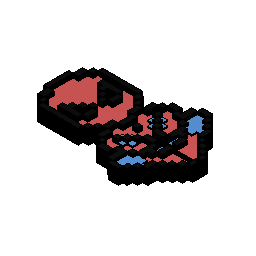
Spider-man v1 (Autodesk Fusion 360 design; units mm, degrees)
Autodesk Fusion 360 part; units mm, degrees
note: some values were not read from the file. Chosen so that the rebuilt part matches the saved one: which bodies a step acts on; which face or edge a step refers to. Set by a fixed rule: which sketch regions a step uses.
sketch "spider-man" plane through (0, 0, 0) normal (0, 0, 1) x (1, 0, 0)
  line L0 (48.5, 2.7143) -> (48.5, 6)
  line L1 (48.5, 6) -> (45.5, 6)
  line L2 (45.5, 6) -> (45.5, 9.5)
  line L3 (45.5, 9.5) -> (42, 9.5)
  line L4 (42, 9.5) -> (42, 13)
  line L5 (42, 13) -> (38.5, 13)
  line L6 (38.5, 13) -> (38.2383, 13)
  line L7 (38.2383, 13) -> (38.2383, 16)
  line L8 (38.2383, 16) -> (35, 16)
  line L9 (35, 16) -> (35, 23)
  line L10 (35, 23) -> (32, 23)
  line L11 (32, 23) -> (32, 26.5)
  line L12 (32, 26.5) -> (28.5, 26.5)
  line L13 (28.5, 26.5) -> (28.5, 30)
  line L14 (28.5, 30) -> (25, 30)
  line L15 (25, 30) -> (25, 33.5)
  line L16 (25, 33.5) -> (18, 33.5)
  line L17 (18, 33.5) -> (18, 30)
  line L18 (18, 30) -> (14, 30)
  line L19 (14, 30) -> (14, 23)
  line L20 (14, 23) -> (11, 23)
  line L21 (11, 23) -> (11, 26.5)
  line L22 (11, 26.5) -> (4.5, 26.5)
  line L23 (4.5, 26.5) -> (4.5, 23)
  line L24 (4.5, 23) -> (1, 23)
  line L25 (1, 23) -> (1, 20)
  line L26 (1, 20) -> (-2.5282, 20)
  line L27 (-2.5282, 20) -> (-2.5282, 13)
  line L28 (-2.5282, 13) -> (-6, 13)
  line L29 (-6, 13) -> (-6, 16.5)
  line L30 (-6, 16.5) -> (-9, 16.5)
  line L31 (-9, 16.5) -> (-9, 20)
  line L32 (-9, 20) -> (-12.5598, 20)
  line L33 (-12.5598, 20) -> (-12.5598, 23)
  line L34 (-12.5598, 23) -> (-40, 23)
  line L35 (-40, 23) -> (-40, 20)
  line L36 (-40, 20) -> (-43.2664, 20)
  line L37 (-43.2664, 20) -> (-43.2664, 16.4387)
  line L38 (-43.2664, 16.4387) -> (-47, 16.4387)
  line L39 (-47, 16.4387) -> (-47, 10)
  line L40 (-47, 10) -> (-50, 10)
  line L41 (-50, 10) -> (-50, -7.0582)
  line L42 (-50, -7.0582) -> (-47, -7.0582)
  line L43 (-47, -7.0582) -> (-47, -14)
  line L44 (-47, -14) -> (-43, -14)
  line L45 (-43, -14) -> (-43, -17.6072)
  line L46 (-43, -17.6072) -> (-40, -17.6072)
  line L47 (-40, -17.6072) -> (-40, -21)
  line L48 (-40, -21) -> (-12.5882, -21)
  line L49 (-12.5882, -21) -> (-12.5882, -17.6072)
  line L50 (-12.5882, -17.6072) -> (-9, -17.6072)
  line L51 (-9, -17.6072) -> (-9, -14.3237)
  line L52 (-9, -14.3237) -> (-6, -14.3237)
  line L53 (-6, -14.3237) -> (-6, -11)
  line L54 (-6, -11) -> (-2.4982, -11)
  line L55 (-2.4982, -11) -> (-2.4982, -18)
  line L56 (-2.4982, -18) -> (1, -18)
  line L57 (1, -18) -> (1, -21)
  line L58 (1, -21) -> (4, -21)
  line L59 (4, -21) -> (4, -25)
  line L60 (4, -25) -> (11.3411, -25)
  line L61 (11.3411, -25) -> (11.3411, -21)
  line L62 (11.3411, -21) -> (14.4254, -21)
  line L63 (14.4254, -21) -> (14.4254, -28)
  line L64 (14.4254, -28) -> (18, -28)
  line L65 (18, -28) -> (18, -31)
  line L66 (18, -31) -> (25, -31)
  line L67 (25, -31) -> (25, -28)
  line L68 (25, -28) -> (28, -28)
  line L69 (28, -28) -> (28, -24)
  line L70 (32, -21) -> (35, -21)
  line L71 (35, -21) -> (35, -14.4641)
  line L72 (35, -14.4641) -> (38.5374, -14.4641)
  line L73 (38.5374, -14.4641) -> (38.5374, -11)
  line L74 (38.5374, -11) -> (42, -11)
  line L75 (42, -11) -> (42, -8)
  line L76 (42, -8) -> (45.5, -8)
  line L77 (45.5, -8) -> (45.5, -4)
  line L78 (48.5, -4) -> (45.5, -4)
  line L79 (48.5, -4) -> (48.5, -0.2857)
  line L80 (48.5, -0.2857) -> (45.5, -0.2857)
  line L81 (45.5, -0.2857) -> (45.5, -4)
  line L82 (45.5, -4) -> (42, -4)
  line L83 (42, -4) -> (42, -8)
  line L84 (38.5439, -8) -> (38.5374, -11)
  line L85 (38.5439, -8) -> (42, -8)
  line L86 (38.5374, -11) -> (35, -11)
  line L87 (35, -11) -> (35, -14.4641)
  line L88 (35, -14.4641) -> (31.5, -14.4641)
  line L89 (31.5, -14.4641) -> (31.5, -21)
  line L90 (31.5, -21) -> (32, -21)
  line L91 (28, -21) -> (28, -24)
  line L92 (31.5, -21) -> (31.5, -24.4721)
  line L93 (31.5, -24.4721) -> (28, -24.4721)
  line L94 (31.5, -21) -> (28, -21)
  line L95 (28, -24.4721) -> (25, -24.4721)
  line L96 (25, -24.4721) -> (25, -28)
  line L97 (25, -28) -> (18, -28)
  line L98 (18, -28) -> (18, -17.6609)
  line L99 (18, -17.6609) -> (21.5, -17.6609)
  line L100 (21.5, -17.6609) -> (21.5, -14.3625)
  line L101 (21.5, -14.3625) -> (25, -14.3625)
  line L102 (25, -14.3625) -> (25, -11)
  line L103 (25, -11) -> (28, -11)
  line L104 (28, -11) -> (28, -7.5019)
  line L105 (28, -7.5019) -> (31.5671, -7.5019)
  line L106 (31.5671, -7.5019) -> (31.5671, -0.2857)
  line L107 (31.5671, -0.2857) -> (28, -0.2857)
  line L108 (28, -0.2857) -> (28, -7.5019)
  line L109 (24.7745, -7.5019) -> (24.7745, -4.1046)
  line L110 (24.7745, -4.1046) -> (21.5, -4.1046)
  line L111 (21.5, -4.1046) -> (21.5, -14.3625)
  line L112 (24.7745, -7.5019) -> (28, -7.5019)
  line L113 (21.5, -4.1046) -> (21.5, -0.6195)
  line L114 (21.5, -0.6195) -> (14.6072, -0.6195)
  line L115 (14.6072, -0.6195) -> (14.6072, -4.1046)
  line L116 (14.6072, -4.1046) -> (21.5, -4.1046)
  line L117 (14.6072, -4.1046) -> (14.6072, -7.4154)
  line L118 (14.6072, -7.4154) -> (11, -7.4154)
  line L119 (11, -7.4154) -> (11, -4.1046)
  line L120 (11, -4.1046) -> (14.6072, -4.1046)
  line L121 (11, -7.4154) -> (11, -11)
  line L122 (11, -11) -> (7.5347, -11)
  line L123 (7.5347, -11) -> (7.5347, -7.4154)
  line L124 (7.5347, -7.4154) -> (11, -7.4154)
  line L125 (7.5347, -11) -> (7.5347, -14)
  line L126 (7.5347, -14) -> (4, -14)
  line L127 (4, -14) -> (4, -11)
  line L128 (4, -11) -> (7.5347, -11)
  line L129 (21.5, -14.3625) -> (18, -14.3625)
  line L130 (18, -14.3625) -> (18, -17.6609)
  line L131 (18, -17.6609) -> (11.3411, -17.6609)
  line L132 (11.3411, -17.6609) -> (11.3411, -21)
  line L133 (11.3411, -21) -> (4, -21)
  line L134 (4, -21) -> (4, -18)
  line L135 (4, -18) -> (1, -18)
  line L136 (1, -18) -> (1, -11)
  line L137 (1, -11) -> (-2.4982, -11)
  line L138 (-2.4982, -11) -> (-2.4982, -4)
  line L139 (-2.4982, -4) -> (1, -4)
  line L140 (1, -4) -> (1, 6)
  line L141 (1, 6) -> (-2.4982, 6)
  line L142 (-2.4982, 6) -> (-2.4982, -4)
  line L143 (-6, -4) -> (-6, -11)
  line L144 (-9, -11) -> (-9, -14.3237)
  line L145 (-9, -14.3237) -> (-12.5882, -14.3237)
  line L146 (-12.5882, -14.3237) -> (-12.5882, -17.6072)
  line L147 (-6, -4) -> (-2.4982, -4)
  line L148 (-9, -11) -> (-6, -11)
  line L149 (7.6928, 2.5546) -> (7.6928, -0.6195)
  line L150 (7.6928, -0.6195) -> (4.3343, -0.6195)
  line L151 (4.3343, -0.6195) -> (4.3343, 2.5546)
  line L152 (4.3343, 2.5546) -> (7.6928, 2.5546)
  line L153 (-12.5882, -17.6072) -> (-40, -17.6072)
  line L154 (-40, -17.6072) -> (-40, -14)
  line L155 (-40, -14) -> (-43, -14)
  line L156 (-43, -14) -> (-43, -7)
  line L157 (-43, -7) -> (-47, -7.0582)
  line L158 (-47, -7.0582) -> (-47, 10)
  line L159 (-47, 10) -> (-43.316, 10)
  line L160 (-43.316, 10) -> (-43.2664, 16.4387)
  line L161 (-43.2664, 16.4387) -> (-40, 16.4387)
  line L162 (-40, 16.4387) -> (-40, 20)
  line L163 (-40, 20) -> (-12.5598, 20)
  line L164 (-12.5598, 20) -> (-12.5598, 16.5)
  line L165 (-12.5598, 16.5) -> (-8.5, 16.5)
  line L166 (-9, 16.5) -> (-9, 13)
  line L167 (-9, 13) -> (-6, 13)
  line L168 (-6, 13) -> (-6, 6)
  line L169 (-6, 6) -> (-2.4982, 6)
  line L170 (-2.4982, 6) -> (-2.5282, 13)
  line L171 (-2.5282, 13) -> (1, 13)
  line L172 (1, 13) -> (1, 20)
  line L173 (1, 20) -> (4.5, 20)
  line L174 (4.5, 20) -> (4.5, 23)
  line L175 (11, 23) -> (11, 20)
  line L176 (11, 20) -> (18, 20)
  line L177 (18, 20) -> (18, 30)
  line L178 (18, 30) -> (25, 30)
  line L179 (25, 30) -> (25, 26.5)
  line L180 (25, 26.5) -> (28.5, 26.5)
  line L181 (28.5, 23) -> (32, 23)
  line L182 (28.5, 23) -> (28.5, 26.5)
  line L183 (32, 23) -> (32, 16)
  line L184 (32, 16) -> (35, 16)
  line L185 (35, 16) -> (35, 13)
  line L186 (35, 13) -> (38.2383, 13)
  line L187 (38.2383, 13) -> (38.2383, 9.5)
  line L188 (38.2383, 9.5) -> (42, 9.5)
  line L189 (42, 9.5) -> (42, 6)
  line L190 (42, 6) -> (45.5, 6)
  line L191 (45.5, 6) -> (45.5, 2.7143)
  line L192 (45.5, 2.7143) -> (48.5, 2.7143)
  line L193 (31.5, 2.7143) -> (31.5, 9.5)
  line L194 (31.5, 9.5) -> (28, 9.5)
  line L195 (28, 9.5) -> (28, 2.7143)
  line L196 (28, 2.7143) -> (31.5, 2.7143)
  line L197 (45.5, 2.7143) -> (31.5, 2.7143)
  line L198 (28, 9.5) -> (25, 9.5)
  line L199 (25, 9.5) -> (25, 2.7741)
  line L200 (25, 2.7741) -> (28, 2.7143)
  line L201 (28, 9.5) -> (28, 13)
  line L202 (28, 13) -> (25, 13)
  line L203 (25, 13) -> (25, 16.2031)
  line L204 (25, 16.2031) -> (21.5, 16.2031)
  line L205 (21.5, 16.2031) -> (21.5, 6.1371)
  line L206 (21.5, 6.1371) -> (25, 6.1371)
  line L207 (21.5, 6.1371) -> (21.5, 2.7741)
  line L208 (21.5, 2.7741) -> (14.5, 2.7741)
  line L209 (14.5, 2.7741) -> (14.5, 6.1371)
  line L210 (14.5, 6.1371) -> (21.5, 6.1371)
  line L211 (14.5, 6.1371) -> (14.5, 9.5)
  line L212 (14.5, 9.5) -> (11, 9.5)
  line L213 (11, 9.5) -> (11, 6.1371)
  line L214 (11, 6.1371) -> (14.5, 6.1371)
  line L215 (14.5, 9.5) -> (14.5, 13)
  line L216 (14.5, 13) -> (11, 13)
  line L217 (11, 13) -> (11, 9.5)
  line L218 (11, 13) -> (11, 16.5)
  line L219 (11, 16.5) -> (7.7586, 16.5)
  line L220 (7.7586, 16.5) -> (7.7586, 13)
  line L221 (7.7586, 13) -> (11, 13)
  line L222 (25, 16.2031) -> (28, 16.2031)
  line L223 (28, 16.2031) -> (28, 19.5)
  line L224 (28, 19.5) -> (32, 19.5)
  line L225 (21.5, 16.2031) -> (21.5, 20)
  line L226 (21.5, 20) -> (18, 20)
  line L227 (18, 20) -> (18, 16.2031)
  line L228 (18, 16.2031) -> (21.5, 16.2031)
  line L229 (7.7586, 16.5) -> (4.5, 16.5)
  line L230 (4.5, 16.5) -> (4.5, 13)
  line L231 (4.5, 13) -> (7.7586, 13)
  line L232 (7.7586, 13) -> (7.7586, 9.5)
  line L233 (7.7586, 9.5) -> (11, 9.5)
  line L234 (7.7586, 9.5) -> (4.5, 9.5)
  line L235 (4.5, 9.5) -> (4.5, 13)
  line L236 (11, 6.1371) -> (7.7586, 6.1371)
  line L237 (7.7586, 6.1371) -> (7.7586, 9.5)
  line L238 (45.5, -0.2857) -> (31.5671, -0.2857)
  line L239 (28, -0.2857) -> (24.7745, -0.2857)
  line L240 (24.7745, -0.2857) -> (24.7745, -4.1046)
  line L241 (25, -14.3625) -> (28, -14.3625)
  line L242 (28, -14.3625) -> (28, -17.5)
  line L243 (28, -17.5) -> (31.5, -17.5)
  line L244 (14.6072, -7.4154) -> (14.6072, -11)
  line L245 (14.6072, -11) -> (11, -11)
  line L246 (11, -11) -> (11, -14)
  line L247 (11, -14) -> (7.5347, -14)
  line L248 (4, -11) -> (4, -7.4154)
  line L249 (4, -7.4154) -> (7.5347, -7.4154)
  line L250 (7.5347, -7.4154) -> (7.5347, -4.1046)
  line L251 (7.5347, -4.1046) -> (11, -4.1046)
  line L252 (-19.5, 13) -> (-16, 13)
  line L253 (-16, 13) -> (-16, 6)
  line L254 (-16, 6) -> (-19.5, 6)
  line L255 (-19.5, 6) -> (-19.5, 13)
  line L256 (-19.5, 13) -> (-19.5, 16.5)
  line L257 (-19.5, 16.5) -> (-33, 16.5)
  line L258 (-33, 16.5) -> (-33, 13)
  line L259 (-33, 13) -> (-30, 13)
  line L260 (-30, 13) -> (-30, 9.5)
  line L261 (-30, 9.5) -> (-26.25, 9.5)
  line L262 (-26.25, 9.5) -> (-26.25, 6)
  line L263 (-26.25, 6) -> (-23, 6)
  line L264 (-23, 6) -> (-23, 2.5)
  line L265 (-23, 2.5) -> (-19.5, 2.5)
  line L266 (-19.5, 2.5) -> (-19.5, 6)
  line L267 (-23, 6) -> (-19.5, 6)
  line L268 (-23, 6) -> (-23, 9.5)
  line L269 (-23, 9.5) -> (-26.25, 9.5)
  line L270 (-26.25, 9.5) -> (-26.25, 13)
  line L271 (-26.25, 13) -> (-19.5, 13)
  line L272 (-19.5, -4) -> (-19.5, -0.5)
  line L273 (-19.5, -0.5) -> (-23, -0.5)
  line L274 (-23, -0.5) -> (-23, -4)
  line L275 (-23, -4) -> (-19.5, -4)
  line L276 (-19.5, -4) -> (-16, -4)
  line L277 (-16, -4) -> (-16, -11)
  line L278 (-16, -11) -> (-19.5, -11)
  line L279 (-19.5, -11) -> (-19.5, -4)
  line L280 (-23, -4) -> (-23, -7.5)
  line L281 (-23, -7.5) -> (-26.5, -7.5)
  line L282 (-26.5, -7.5) -> (-26.5, -4)
  line L283 (-26.5, -4) -> (-23, -4)
  line L284 (-26.5, -7.5) -> (-26.5, -11)
  line L285 (-26.5, -11) -> (-19.5, -11)
  line L286 (-19.5, -14.5) -> (-33, -14.5)
  line L287 (-33, -14.5) -> (-33, -11)
  line L288 (-33, -11) -> (-30, -11)
  line L289 (-30, -11) -> (-30, -7.5)
  line L290 (-30, -7.5) -> (-26.5, -7.5)
  line L291 (48.5, 2.7143) -> (48.5, -0.2857)
  line L292 (45.5, -0.2857) -> (45.5, 2.7143)
  line L293 (-19.5, -14.5) -> (-19.5, -11)
  line L294 (4.5, 23) -> (11, 23)
  line L295 (18.0536, -0.6195) -> (18, 2.7741)
  circle A0 centre (47, 1.1917) radius 1.2764
  constraint vertical L0
  constraint perpendicular L0 L1
  constraint perpendicular L1 L2
  constraint perpendicular L2 L3
  constraint perpendicular L3 L4
  constraint perpendicular L4 L5
  constraint parallel L5 L6
  constraint perpendicular L6 L7
  constraint perpendicular L7 L8
  constraint perpendicular L6 L9
  constraint perpendicular L9 L10
  constraint perpendicular L10 L11
  constraint perpendicular L11 L12
  constraint perpendicular L12 L13
  constraint perpendicular L13 L14
  constraint perpendicular L14 L15
  constraint perpendicular L15 L16
  constraint perpendicular L16 L17
  constraint perpendicular L17 L18
  constraint perpendicular L18 L19
  constraint perpendicular L19 L20
  constraint perpendicular L20 L21
  constraint perpendicular L21 L22
  constraint perpendicular L22 L23
  constraint perpendicular L23 L24
  constraint perpendicular L24 L25
  constraint perpendicular L25 L26
  constraint perpendicular L26 L27
  constraint perpendicular L27 L28
  constraint perpendicular L28 L29
  constraint perpendicular L29 L30
  constraint perpendicular L28 L31
  constraint perpendicular L31 L32
  constraint perpendicular L32 L33
  constraint perpendicular L33 L34
  constraint perpendicular L34 L35
  constraint perpendicular L35 L36
  constraint perpendicular L36 L37
  constraint perpendicular L37 L38
  constraint perpendicular L38 L39
  constraint perpendicular L39 L40
  constraint perpendicular L40 L41
  constraint perpendicular L41 L42
  constraint perpendicular L42 L43
  constraint perpendicular L43 L44
  constraint perpendicular L44 L45
  constraint perpendicular L45 L46
  constraint perpendicular L46 L47
  constraint perpendicular L47 L48
  constraint perpendicular L48 L49
  constraint perpendicular L49 L50
  constraint perpendicular L50 L51
  constraint perpendicular L51 L52
  constraint perpendicular L52 L53
  constraint perpendicular L53 L54
  constraint perpendicular L54 L55
  constraint perpendicular L55 L56
  constraint perpendicular L56 L57
  constraint perpendicular L57 L58
  constraint perpendicular L58 L59
  constraint perpendicular L59 L60
  constraint perpendicular L58 L61
  constraint perpendicular L61 L62
  constraint perpendicular L62 L63
  constraint perpendicular L63 L64
  constraint perpendicular L64 L65
  constraint perpendicular L65 L66
  constraint perpendicular L66 L67
  constraint perpendicular L67 L68
  constraint perpendicular L68 L69
  constraint perpendicular L71 L72
  constraint perpendicular L72 L73
  constraint perpendicular L73 L74
  constraint perpendicular L72 L75
  constraint perpendicular L75 L76
  constraint perpendicular L76 L77
  constraint perpendicular L77 L78
  constraint perpendicular L78 L79
  constraint perpendicular L79 L80
  constraint perpendicular L78 L81
  constraint perpendicular L77 L82
  constraint perpendicular L76 L83
  constraint perpendicular L75 L85
  constraint perpendicular L73 L86
  constraint perpendicular L72 L87
  constraint perpendicular L71 L88
  constraint perpendicular L88 L89
  constraint perpendicular L90 L92
  constraint coincident L69 L93.end
  constraint perpendicular L69 L93
  constraint perpendicular L92 L94
  constraint perpendicular L69 L95
  constraint perpendicular L68 L96
  constraint perpendicular L65 L97
  constraint perpendicular L97 L98
  constraint perpendicular L98 L99
  constraint perpendicular L99 L100
  constraint perpendicular L100 L101
  constraint perpendicular L101 L102
  constraint perpendicular L102 L103
  constraint perpendicular L103 L104
  constraint perpendicular L104 L105
  constraint perpendicular L105 L106
  constraint perpendicular L106 L107
  constraint perpendicular L105 L108
  constraint perpendicular L105 L109
  constraint perpendicular L109 L110
  constraint perpendicular L101 L111
  constraint perpendicular L104 L112
  constraint perpendicular L110 L113
  constraint perpendicular L113 L114
  constraint perpendicular L114 L115
  constraint perpendicular L111 L116
  constraint perpendicular L116 L117
  constraint perpendicular L117 L118
  constraint perpendicular L118 L119
  constraint perpendicular L117 L120
  constraint perpendicular L118 L121
  constraint perpendicular L121 L122
  constraint perpendicular L122 L123
  constraint perpendicular L121 L124
  constraint perpendicular L122 L125
  constraint perpendicular L123 L126
  constraint perpendicular L126 L127
  constraint perpendicular L123 L128
  constraint perpendicular L100 L129
  constraint perpendicular L99 L130
  constraint perpendicular L98 L131
  constraint perpendicular L62 L132
  constraint perpendicular L59 L133
  constraint perpendicular L58 L134
  constraint perpendicular L59 L135
  constraint perpendicular L135 L136
  constraint perpendicular L55 L137
  constraint perpendicular L54 L138
  constraint perpendicular L138 L139
  constraint perpendicular L139 L140
  constraint perpendicular L140 L141
  constraint perpendicular L139 L142
  constraint perpendicular L54 L143
  constraint perpendicular L52 L144
  constraint perpendicular L144 L145
  constraint perpendicular L50 L146
  constraint perpendicular L142 L147
  constraint perpendicular L143 L148
  constraint vertical L149
  constraint perpendicular L149 L150
  constraint perpendicular L150 L151
  constraint perpendicular L149 L152
  constraint perpendicular L47 L153
  constraint perpendicular L153 L154
  constraint perpendicular L45 L155
  constraint perpendicular L155 L156
  constraint perpendicular L40 L158
  constraint perpendicular L158 L159
  constraint perpendicular L37 L161
  constraint perpendicular L36 L162
  constraint perpendicular L33 L163
  constraint perpendicular L163 L164
  constraint coincident L30 L165.end
  constraint perpendicular L164 L165
  constraint perpendicular L165 L166
  constraint perpendicular L29 L167
  constraint perpendicular L167 L168
  constraint perpendicular L142 L169
  constraint perpendicular L26 L172
  constraint perpendicular L172 L173
  constraint perpendicular L24 L174
  constraint perpendicular L20 L175
  constraint perpendicular L175 L176
  constraint perpendicular L18 L177
  constraint perpendicular L15 L178
  constraint perpendicular L14 L179
  constraint perpendicular L13 L180
  constraint perpendicular L11 L181
  constraint perpendicular L180 L182
  constraint perpendicular L181 L183
  constraint perpendicular L9 L184
  constraint perpendicular L8 L185
  constraint perpendicular L7 L186
  constraint perpendicular L6 L187
  constraint perpendicular L4 L188
  constraint perpendicular L188 L189
  constraint perpendicular L2 L190
  constraint perpendicular L1 L191
  constraint perpendicular L0 L192
  constraint vertical L193
  constraint perpendicular L193 L194
  constraint perpendicular L194 L195
  constraint perpendicular L193 L196
  constraint perpendicular L193 L197
  constraint perpendicular L195 L198
  constraint perpendicular L198 L199
  constraint perpendicular L198 L201
  constraint perpendicular L201 L202
  constraint perpendicular L198 L203
  constraint perpendicular L201 L204
  constraint perpendicular L204 L205
  constraint midpoint L199 L206.end
  constraint perpendicular L199 L206
  constraint perpendicular L206 L207
  constraint perpendicular L205 L208
  constraint perpendicular L208 L209
  constraint perpendicular L205 L210
  constraint perpendicular L210 L211
  constraint perpendicular L211 L212
  constraint perpendicular L210 L213
  constraint perpendicular L211 L214
  constraint perpendicular L212 L215
  constraint perpendicular L215 L216
  constraint perpendicular L212 L217
  constraint perpendicular L216 L218
  constraint perpendicular L218 L219
  constraint perpendicular L216 L220
  constraint perpendicular L217 L221
  constraint perpendicular L203 L222
  constraint perpendicular L222 L223
  constraint midpoint L183 L224.end
  constraint perpendicular L183 L224
  constraint perpendicular L204 L225
  constraint perpendicular L177 L226
  constraint perpendicular L176 L227
  constraint perpendicular L205 L228
  constraint perpendicular L220 L229
  constraint perpendicular L229 L230
  constraint perpendicular L220 L231
  constraint perpendicular L231 L232
  constraint perpendicular L213 L233
  constraint perpendicular L232 L234
  constraint perpendicular L231 L235
  constraint perpendicular L213 L236
  constraint perpendicular L233 L237
  constraint perpendicular L108 L239
  constraint perpendicular L110 L240
  constraint perpendicular L102 L241
  constraint perpendicular L241 L242
  constraint coincident L89 L243.end
  constraint perpendicular L89 L243
  constraint perpendicular L118 L244
  constraint perpendicular L121 L245
  constraint perpendicular L245 L246
  constraint perpendicular L125 L247
  constraint perpendicular L128 L248
  constraint perpendicular L248 L249
  constraint perpendicular L249 L250
  constraint perpendicular L250 L251
  constraint perpendicular L31 L252
  constraint perpendicular L252 L253
  constraint perpendicular L31 L254
  constraint perpendicular L252 L255
  constraint perpendicular L252 L256
  constraint perpendicular L255 L257
  constraint perpendicular L257 L258
  constraint perpendicular L258 L259
  constraint perpendicular L257 L260
  constraint perpendicular L258 L261
  constraint perpendicular L261 L262
  constraint perpendicular L258 L263
  constraint perpendicular L261 L264
  constraint perpendicular L258 L265
  constraint perpendicular L254 L266
  constraint perpendicular L266 L267
  constraint perpendicular L267 L268
  constraint perpendicular L262 L269
  constraint perpendicular L261 L270
  constraint perpendicular L256 L271
  constraint vertical L272
  constraint perpendicular L272 L273
  constraint perpendicular L273 L274
  constraint perpendicular L272 L275
  constraint perpendicular L272 L276
  constraint perpendicular L276 L277
  constraint perpendicular L277 L278
  constraint perpendicular L275 L279
  constraint perpendicular L275 L280
  constraint perpendicular L280 L281
  constraint perpendicular L281 L282
  constraint perpendicular L280 L283
  constraint perpendicular L281 L284
  constraint perpendicular L279 L285
  constraint perpendicular L279 L286
  constraint perpendicular L278 L287
  constraint perpendicular L287 L288
  constraint perpendicular L288 L289
  constraint perpendicular L282 L290
  constraint perpendicular L80 L291
  constraint perpendicular L192 L292
  constraint perpendicular L81 L238
  constraint perpendicular L285 L293
  constraint perpendicular L21 L294
  constraint midpoint L114 L295.start
  constraint midpoint L208 L295.end
extrude "Extrude1" add sketch "spider-man" along normal blind 7 contours L183 L184 L185 L186 L187 L188 L189 L190 L191 L193 L194 L197 L201 L202 L203 L222 L223 L224 | L81 L82 L83 L84 L85 L86 L87 L88 L89 L102 L103 L104 L105 L106 L238 L241 L242 L243 | L111 L114 L115 L116 L129 L130 L131 L132 L133 L134 L135 L136 L137 L138 L139 L140 L141 L170 L171 L172 L173 L174 L175 L176 L205 L208 L209 L210 L227 L228 L294 L295 | L142 L143 L144 L145 L146 L147 L148 L153 L154 L155 L156 L157 L158 L159 L160 L161 L162 L163 L164 L165 L166 L167 L168 L169 makes body 1 at (-38.772, 4.1667, 0) makes body 1 at (16.8333, 8.4247, 7) makes body 2 at (33.7461, 7.2381, 0) makes body 3 at (33.8927, -5.2625, 0)
extrude "Extrude2" add sketch "spider-man" along normal blind 10 separate body contours L0 L1 L191 L192 | L80 L192 L291 L292 | L78 L79 L80 L81 | L2 L3 L189 L190 | L193 L194 L195 L196 | L76 L77 L82 L83 | L105 L106 L107 L108 | L4 L5 L6 L187 L188 | L198 L199 L201 L202 L203 L204 L205 L206 | L74 L75 L84 L85 | L101 L102 L103 L104 L109 L110 L111 L112 | L7 L8 L185 L186 | L117 L118 L119 L120 | L211 L212 L213 L214 | L207 L208 L209 L210 | L225 L226 L227 L228 | L72 L73 L86 L87 | L113 L114 L115 L116 | L9 L10 L183 L184 | L99 L100 L129 L130 | L18 L19 L20 L175 L176 L177 | L217 L221 L232 L233 | L70 L71 L88 L89 L90 | L11 L12 L181 L182 | L15 L16 L17 L178 | L62 L63 L64 L98 L131 L132 | L121 L122 L123 L124 | L21 L22 L23 L294 | L13 L14 L179 L180 | L220 L229 L230 L231 | L65 L66 L67 L97 | L24 L25 L173 L174 | L69 L91 L92 L93 L94 | L68 L69 L95 L96 | L59 L60 L61 L133 | L125 L126 L127 L128 | L57 L58 L134 L135 | L26 L27 L171 L172 | L55 L56 L136 L137 | L28 L168 L169 L170 | L29 L30 L165 L166 L167 | L139 L140 L141 L142 | L54 L138 L143 L147 | L52 L53 L144 L148 | L31 L32 L164 L165 | L50 L51 L145 L146 | L33 L34 L35 L163 | L36 L37 L161 L162 | L47 L48 L49 L153 | L45 L46 L154 L155 | L38 L39 L159 L160 | L43 L44 L156 L157 | L40 L41 L42 L158 | L149 L150 L151 L152 | L252 L253 L254 L255 | L256 L257 L258 L259 L260 L261 L270 L271 | L264 L265 L266 L267 | L262 L263 L268 L269 | L272 L273 L274 L275 | L276 L277 L278 L279 | L280 L281 L282 L283 | L284 L285 L286 L287 L288 L289 L290 L293 makes body 4 at (-47, -1.3722, 3.3333) makes body 4 at (-43, -11.6667, 3.3333) makes body 4 at (-43.2995, 12.1462, 3.3333) makes body 4 at (-43, -15.2024, 3.3333) makes body 4 at (-43.2664, 18.8129, 3.3333) makes body 4 at (-21.7254, -17.6072, 3.3333) makes body 4 at (-30.8533, 20, 3.3333) makes body 4 at (-11.3921, -17.6072, 3.3333) makes body 4 at (-10.1866, 20, 3.3333) makes body 4 at (-9, -12.1079, 3.3333) makes body 4 at (-9, 15.3333, 3.3333) makes body 4 at (-6, -6.3333, 3.3333) makes body 4 at (-2.5082, 8.3333, 6.6667) makes body 4 at (-2.4982, -13.3333, 3.3333) makes body 4 at (-2.5282, 17.6667, 3.3333) makes body 4 at (-2.4982, 2.6667, 3.3333) makes body 4 at (1, -19, 3.3333) makes body 4 at (2.1667, 20, 3.3333) makes body 4 at (8.8941, -21, 3.3333) makes body 4 at (6.6667, 23, 3.3333) makes body 4 at (18, -24.5536, 3.3333) makes body 4 at (18, 23.3333, 3.3333) makes body 4 at (19.1667, -17.6609, 3.3333) makes body 4 at (18, 18.7344, 3.3333) makes body 4 at (22.6667, -28, 3.3333) makes body 4 at (22.6667, 33.5, 3.3333) makes body 4 at (25, -25.648, 3.3333) makes body 4 at (21.5, -7.5239, 3.3333) makes body 4 at (27.3333, 30, 3.3333) makes body 4 at (21.5, 12.8478, 3.3333) makes body 4 at (16.9048, -4.1046, 3.3333) makes body 4 at (16.8333, 6.1371, 3.3333) makes body 4 at (30.3333, -24.4721, 3.3333) makes body 4 at (12.2024, -4.1046, 6.6667) makes body 4 at (28.5, 24.1667, 3.3333) makes body 4 at (12.1667, 6.1371, 3.3333) makes body 4 at (28, -2.6911, 3.3333) makes body 4 at (28, 7.2381, 3.3333) makes body 4 at (31.5, -16.6427, 3.3333) makes body 4 at (7.5347, -9.8051, 3.3333) makes body 4 at (32, 20.6667, 3.3333) makes body 4 at (7.7586, 11.8333, 3.3333) makes body 4 at (5.1782, -14, 6.6667) makes body 4 at (37.1589, 16, 3.3333) makes body 4 at (4.5, 15.3333, 3.3333) makes body 4 at (36.1791, -14.4641, 3.3333) makes body 4 at (40.7461, 13, 3.3333) makes body 4 at (39.6916, -11, 3.3333) makes body 4 at (42, 8.3333, 3.3333) makes body 4 at (45.5, -6.6667, 3.3333) makes body 4 at (48.5, -0.6667, 3.3333) makes body 5 at (-24, -14.5, 3.3333) makes body 5 at (-16, -6.3333, 3.3333) makes body 5 at (-21.8333, -4, 3.3333) makes body 5 at (-24.1667, -7.5, 3.3333) makes body 6 at (-26.25, 8.3333, 3.3333) makes body 6 at (-23, 4.8333, 3.3333) makes body 6 at (-24, 16.5, 3.3333) makes body 6 at (-16, 10.6667, 3.3333) makes body 7 at (6.5733, -0.6195, 3.3333)
extrude "Extrude3" add sketch "spider-man" along normal blind 4 separate body contours L80 L192 L291 L292 | A0 makes body 8
combine "Combine1" operation add target body 4 tool bodies 5 6 7 8 makes body 10 at (6.5733, -0.6195, 3.3333) makes body 9 at (-24, -14.5, 3.3333) makes body 9 at (-16, -6.3333, 3.3333) makes body 9 at (-21.8333, -4, 3.3333) makes body 9 at (-24.1667, -7.5, 3.3333) makes body 11 at (-26.25, 8.3333, 3.3333) makes body 11 at (-23, 4.8333, 3.3333) makes body 11 at (-24, 16.5, 3.3333) makes body 11 at (-16, 10.6667, 3.3333)
extrude "Extrude4" add sketch "spider-man" along normal blind 8 separate body contours L195 L198 L199 L200 | L108 L109 L112 L239 L240 | L177 L178 L179 L180 L181 L182 L183 L204 L222 L223 L224 L225 L226 | L212 L215 L216 L217 | L213 L233 L236 L237 | L69 L89 L91 L94 L95 L96 L97 L98 L99 L100 L101 L241 L242 L243 | L118 L121 L244 L245 | L119 L124 L250 L251 | L218 L219 L220 L221 | L231 L232 L234 L235 | L122 L125 L246 L247 | L123 L128 L248 L249 makes body 13 at (7.7586, 11.8333, 2.6667) makes body 13 at (7.7586, 7.258, 2.6667) makes body 13 at (7.7586, 15.3333, 2.6667) makes body 13 at (13.3333, 9.5, 2.6667) makes body 14 at (8.6898, -7.4154, 2.6667) makes body 14 at (13.4048, -11, 2.6667) makes body 14 at (7.5347, -9.8051, 2.6667) makes body 14 at (9.8449, -11, 2.6667) makes body 16 at (28, -2.6911, 2.6667) makes body 12 at (28, 7.2381, 5.3333) makes body 15 at (21.5, 25.5, 0) makes body 17 at (21.5, -23.3776, 0)
combine "Combine2" operation add target body 12 tool bodies 13 14 15 16 17 makes body 21 at (21.5, 25.5, 0) makes body 19 at (28, -2.6911, 2.6667) makes body 22 at (21.5, -23.3776, 0) makes body 20 at (7.7586, 11.8333, 2.6667) makes body 20 at (7.7586, 7.258, 2.6667) makes body 20 at (7.7586, 15.3333, 2.6667) makes body 20 at (13.3333, 9.5, 2.6667) makes body 18 at (8.6898, -7.4154, 2.6667) makes body 18 at (13.4048, -11, 2.6667) makes body 18 at (7.5347, -9.8051, 2.6667) makes body 18 at (9.8449, -11, 2.6667)
combine "Combine3" operation add target body 2 tool bodies 22 21 20 19 18 12 11 10 9 4 3 1
hole "Hole1" at (46.9753, 1.1917, 4) direction (0, 0, -1) diameter 2.4 depth 4.8 tip angle 180 countersink diameter 2.6 countersink angle 90 bodies 2
named bodies: "red", "outline", "right eye", "middle dot", "left eye", "left foot", "right squares", "right foot", "left squares", "left leg", "right leg", "spider-man", "red right leg"
